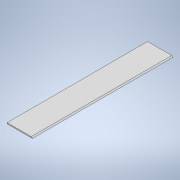
# Autodesk Inventor part: BLADE
Saved by Autodesk Inventor 2020 (Build 240168000, 168)
## iProperties
Created: 2019-11-06
Part Number: BLADE
Material: Generic
Document SubType Name: Modeling
Designer: atmat
Density: 1 g/cm^3
Appearance: Default
Author: atmat
Autodesk Inventor part; units mm, degrees
ref_plane "YZ Plane" through (0, 0, 0) normal (1, 0, 0) x (0, 1, 0)
ref_plane "XZ Plane" through (0, 0, 0) normal (0, 1, 0) x (-1, 0, 0)
ref_plane "XY Plane" through (0, 0, 0) normal (0, 0, 1) x (1, 0, 0)
sketch "Sketch1" plane through (0, 0, 0) normal (0, 1, 0) x (-1, 0, 0)
  line L0 (90, 500) -> (-90, 500)
  line L1 (-90, 500) -> (-90, -500)
  line L2 (-90, -500) -> (90, -500)
  line L3 (90, -500) -> (90, 500)
  point P0 (0, 0)
  dimension "d0" = 180
  dimension "d1" = 90
  dimension "d2" = 1000
  dimension "d3" = 500
  constraints: 8 end point, 2 parallel, 1 horizontal, 1 perpendicular
  measures "d0" distance of L0.start L0.end
  measures "d1" distance from line of L3 point (0, 0)
  measures "d2" distance of L2.end L0.start
  measures "d3" distance from line of point (0, 0) L0
extrude "Extrusion1" add sketch "Sketch1" along normal blind 8
chamfer "Chamfer1" distance 8 angle 45 1 edges at (90, 8, 0)
body "Solid1"
